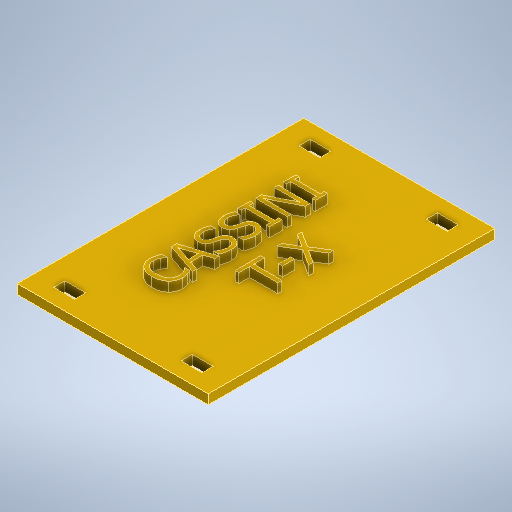
# Autodesk Inventor part: au-dessus hélice
Saved by Autodesk Inventor 2026.2 (Build 302298010, 298A)
## iProperties
Created: 2026-04-02
Part Number: au-dessus hélice
Material: Générique
Document SubType Name: Modeling
Designer: Genon
Density: 1 g/cm^3
Appearance: Or
Author: Genon
Autodesk Inventor part; units mm, degrees
ref_plane "YZ Plane" through (0, 0, 0) normal (1, 0, 0) x (0, 1, 0)
ref_plane "XZ Plane" through (0, 0, 0) normal (0, 1, 0) x (-1, 0, 0)
ref_plane "XY Plane" through (0, 0, 0) normal (0, 0, 1) x (1, 0, 0)
sketch "Esquisse1" plane through (0, 0, 0) normal (0, 1, 0) x (-1, 0, 0)
  line L0 (0, 0) -> (60, 0)
  line L1 (60, 0) -> (60, -90)
  line L2 (60, -90) -> (0, -90)
  line L3 (0, -90) -> (0, 0)
  dimension "d0" = 60
  dimension "d1" = 90
  constraints: 8 end point, 2 parallel, 1 horizontal, 1 perpendicular
  measures "d0" distance of L1.end L2.end
  measures "d1" distance of L0.end L1.end
extrude "Extrusion1" add sketch "Esquisse1" along normal blind 3
sketch "Esquisse3" plane through (0, 3, 0) normal (0, 1, 0) x (1, 0, 0)
  line L0 (-60, 0) -> (0, 0) projected
  line L1 (-30, 0) -> (-30, 90)
  line L2 (0, 90) -> (-60, 90) projected
  line L3 (-30, 45) -> (-60, 45)
  line L4 (-60, 0) -> (-60, 5)
  line L5 (-60, 90) -> (-60, 0) projected
  line L6 (-60, 5) -> (-53, 5)
  line L7 (-53, 5) -> (-47, 5)
  line L8 (-47, 5) -> (-47, 8)
  line L9 (-47, 8) -> (-53, 8)
  line L10 (-53, 8) -> (-53, 5)
  line L11 (-53, 85) -> (-47, 85)
  line L12 (-47, 85) -> (-47, 82)
  line L13 (-47, 82) -> (-53, 82)
  line L14 (-53, 82) -> (-53, 85)
  line L15 (-7, 5) -> (-13, 5)
  line L16 (-13, 5) -> (-13, 8)
  line L17 (-13, 8) -> (-7, 8)
  line L18 (-7, 8) -> (-7, 5)
  line L19 (-7, 82) -> (-7, 85)
  line L20 (-13, 82) -> (-7, 82)
  line L21 (-7, 85) -> (-13, 85)
  line L22 (-13, 85) -> (-13, 82)
  line L23 (-53, 8) -> (-53.25, 8)
  line L24 (-53.25, 8) -> (-53.25, 4.75)
  line L25 (-53.25, 4.75) -> (-53, 4.75)
  line L26 (-53, 4.75) -> (-53, 8)
  line L27 (-47, 4.75) -> (-46.75, 4.75)
  line L28 (-46.75, 4.75) -> (-46.75, 8.25)
  line L29 (-46.75, 8.25) -> (-47, 8.25)
  line L30 (-47, 8.25) -> (-47, 4.75)
  line L31 (-47, 8.25) -> (-53.25, 8.25)
  line L32 (-53.25, 8.25) -> (-53.25, 8)
  line L33 (-53.25, 8) -> (-47, 8)
  line L34 (-47, 8) -> (-47, 8.25)
  line L35 (-53, 4.75) -> (-47, 4.75)
  line L36 (-47, 4.75) -> (-47, 5)
  line L37 (-47, 5) -> (-53, 5)
  line L38 (-53, 5) -> (-53, 4.75)
  line L39 (-53.25, 82) -> (-53.25, 85.25)
  line L40 (-53.25, 85.25) -> (-53, 85.25)
  line L41 (-47, 85.25) -> (-46.75, 85.25)
  line L42 (-46.75, 85.25) -> (-46.75, 81.75)
  line L43 (-46.75, 81.75) -> (-47, 81.75)
  line L44 (-47, 81.75) -> (-53.25, 81.75)
  line L45 (-53.25, 81.75) -> (-53.25, 82)
  line L46 (-53, 85.25) -> (-47, 85.25)
  line L47 (-6.75, 8) -> (-6.75, 4.75)
  line L48 (-6.75, 4.75) -> (-7, 4.75)
  line L49 (-13, 4.75) -> (-13.25, 4.75)
  line L50 (-13.25, 4.75) -> (-13.25, 8.25)
  line L51 (-13.25, 8.25) -> (-13, 8.25)
  line L52 (-13, 8.25) -> (-6.75, 8.25)
  line L53 (-6.75, 8.25) -> (-6.75, 8)
  line L54 (-7, 4.75) -> (-13, 4.75)
  line L55 (-6.75, 82) -> (-6.75, 85.25)
  line L56 (-6.75, 81.75) -> (-6.75, 82)
  line L57 (-13, 81.75) -> (-6.75, 81.75)
  line L58 (-13.25, 81.75) -> (-13, 81.75)
  line L59 (-13.25, 85.25) -> (-13.25, 81.75)
  line L60 (-13, 85.25) -> (-13.25, 85.25)
  line L61 (-7, 85.25) -> (-13, 85.25)
  line L62 (-6.75, 85.25) -> (-7, 85.25)
  dimension "d13" = 5
  dimension "d14" = 7
  dimension "d15" = 6
  dimension "d16" = 3
  dimension "d21" = 0.25
  dimension "d22" = 3.25
  dimension "d23" = 0.25
  dimension "d24" = 3.5
  constraints: 120 end point, 39 symmetric about line, 8 parallel, 8 perpendicular, 6 point on line, 5 horizontal, 3 midpoint
  measures "d13" distance of L0.start L4.end
  measures "d14" distance of L4.end L6.end
  measures "d15" distance of L6.end L7.end
  measures "d16" distance of L7.end L8.end
  measures "d21" distance of L25.end L24.end
  measures "d22" distance of L24.end L23.end
  measures "d23" distance of L29.end L28.end
  measures "d24" distance of L28.end L27.end
extrude "Extrusion2" cut sketch "Esquisse3" against normal through all contours L24 L23 L10 L6 | L6 L26 L25 L24 | L10 L9 L8 L7 | L7 L30 L35 L26 | L32 L31 L30 L9 L23 | L8 L30 L29 L28 L27 | L11 L12 L13 L14 | L15 L16 L17 L18 | L20 L22 L21 L19 | L39 L40 L46 L41 L42 L43 L44 L45 | L47 L48 L54 L49 L50 L51 L52 L53 | L56 L57 L58 L59 L60 L61 L62 L55
sketch "Esquisse4" plane through (0, 3, 0) normal (0, 1, 0) x (1, 0, 0)
  line L0 (-45.4887, 21.9491) -> (-45.4887, 68.6531) construction
  line L1 (-45.4887, 68.6531) -> (-13.8502, 68.6531) construction
  line L2 (-13.8502, 68.6531) -> (-13.8502, 21.9491) construction
  line L3 (-13.8502, 21.9491) -> (-45.4887, 21.9491) construction
  spline S0 degree 2 poles (-32.6344, 24.588) (-32.6344, 23.6155) (-33.2908, 21.9705) (-33.9472, 21.3708) knots 0 0 0 1 2 2 2
  spline S1 degree 2 poles (-33.9472, 21.3708) (-34.5955, 20.7711) (-36.5404, 20.1147) (-37.8045, 20.1147) knots 0 0 0 1 2 2 2
  spline S2 degree 2 poles (-37.8045, 20.1147) (-39.0606, 20.1147) (-40.9245, 20.7549) (-41.6133, 21.3627) knots 0 0 0 1 2 2 2
  spline S3 degree 2 poles (-41.6133, 21.3627) (-42.2859, 21.9624) (-42.9909, 23.5993) (-42.9909, 24.6123) knots 0 0 0 1 2 2 2
  spline S4 degree 2 poles (-42.9909, 24.6123) (-42.9909, 25.1147) (-42.8451, 25.998) (-42.7316, 26.3708) knots 0 0 0 1 2 2 2
  spline S5 degree 2 poles (-42.7316, 26.3708) (-42.6263, 26.6949) (-42.3264, 27.3675) (-42.1481, 27.6998) knots 0 0 0 1 2 2 2
  line L4 (-42.1481, 27.6998) -> (-40.5436, 27.6998)
  line L5 (-40.5436, 27.6998) -> (-40.5436, 27.5945)
  spline S6 degree 2 poles (-40.5436, 27.5945) (-40.7057, 27.4162) (-41.1595, 26.8651) (-41.3783, 26.468) knots 0 0 0 1 2 2 2
  spline S7 degree 2 poles (-41.3783, 26.468) (-41.589, 26.0872) (-41.8564, 25.1876) (-41.8564, 24.6042) knots 0 0 0 1 2 2 2
  spline S8 degree 2 poles (-41.8564, 24.6042) (-41.8564, 23.964) (-41.3297, 22.8214) (-40.8272, 22.3919) knots 0 0 0 1 2 2 2
  spline S9 degree 2 poles (-40.8272, 22.3919) (-40.3167, 21.9705) (-38.7689, 21.5005) (-37.8045, 21.5005) knots 0 0 0 1 2 2 2
  spline S10 degree 2 poles (-37.8045, 21.5005) (-36.7754, 21.5005) (-35.2924, 21.9948) (-34.7819, 22.4243) knots 0 0 0 1 2 2 2
  spline S11 degree 2 poles (-34.7819, 22.4243) (-34.2875, 22.8457) (-33.7851, 23.9721) (-33.7851, 24.6042) knots 0 0 0 1 2 2 2
  spline S12 degree 2 poles (-33.7851, 24.6042) (-33.7851, 25.1795) (-34.0687, 26.1601) (-34.2794, 26.541) knots 0 0 0 1 2 2 2
  spline S13 degree 2 poles (-34.2794, 26.541) (-34.4901, 26.9056) (-34.9277, 27.4486) (-35.0817, 27.6026) knots 0 0 0 1 2 2 2
  line L6 (-35.0817, 27.6026) -> (-35.0817, 27.6998)
  line L7 (-35.0817, 27.6998) -> (-33.4934, 27.6998)
  spline S14 degree 2 poles (-33.4934, 27.6998) (-33.3394, 27.3675) (-33.0558, 26.7841) (-32.9261, 26.3708) knots 0 0 0 1 2 2 2
  spline S15 degree 2 poles (-32.9261, 26.3708) (-32.7802, 25.9332) (-32.6344, 25.1876) (-32.6344, 24.588) knots 0 0 0 1 2 2 2
  line L8 (-32.8127, 27.8619) -> (-42.8127, 31.233)
  line L9 (-42.8127, 31.233) -> (-42.8127, 32.87)
  line L10 (-42.8127, 32.87) -> (-32.8127, 36.2411)
  line L11 (-32.8127, 36.2411) -> (-32.8127, 34.8392)
  line L12 (-32.8127, 34.8392) -> (-35.6084, 33.9316)
  line L13 (-35.6084, 33.9316) -> (-35.6084, 30.1147)
  line L14 (-35.6084, 30.1147) -> (-32.8127, 29.2071)
  line L15 (-32.8127, 29.2071) -> (-32.8127, 27.8619)
  line L16 (-36.743, 33.5669) -> (-41.4512, 32.0191)
  line L17 (-41.4512, 32.0191) -> (-36.743, 30.4794)
  line L18 (-36.743, 30.4794) -> (-36.743, 33.5669)
  spline S16 degree 2 poles (-32.6344, 39.9769) (-32.6344, 38.891) (-33.0882, 37.3675) (-33.4123, 36.6949) knots 0 0 0 1 2 2 2
  line L19 (-33.4123, 36.6949) -> (-35.0817, 36.6949)
  line L20 (-35.0817, 36.6949) -> (-35.0817, 36.7922)
  spline S17 degree 2 poles (-35.0817, 36.7922) (-34.4658, 37.4486) (-33.7851, 39.1099) (-33.7851, 39.8797) knots 0 0 0 1 2 2 2
  spline S18 degree 2 poles (-33.7851, 39.8797) (-33.7851, 40.9818) (-34.7008, 42.1082) (-35.4545, 42.1082) knots 0 0 0 1 2 2 2
  spline S19 degree 2 poles (-35.4545, 42.1082) (-36.0541, 42.1082) (-36.7997, 41.5167) (-36.9861, 40.8765) knots 0 0 0 1 2 2 2
  spline S20 degree 2 poles (-36.9861, 40.8765) (-37.1157, 40.4146) (-37.294, 39.6447) (-37.4399, 39.0693) knots 0 0 0 1 2 2 2
  spline S21 degree 2 poles (-37.4399, 39.0693) (-37.5776, 38.5507) (-37.9909, 37.7322) (-38.3232, 37.4162) knots 0 0 0 1 2 2 2
  spline S22 degree 2 poles (-38.3232, 37.4162) (-38.6554, 37.1082) (-39.5468, 36.7679) (-40.1303, 36.7679) knots 0 0 0 1 2 2 2
  spline S23 degree 2 poles (-40.1303, 36.7679) (-41.3459, 36.7679) (-42.9909, 38.6641) (-42.9909, 40.1309) knots 0 0 0 1 2 2 2
  spline S24 degree 2 poles (-42.9909, 40.1309) (-42.9909, 40.9737) (-42.6587, 42.4648) (-42.3426, 43.105) knots 0 0 0 1 2 2 2
  line L21 (-42.3426, 43.105) -> (-40.7543, 43.105)
  line L22 (-40.7543, 43.105) -> (-40.7543, 43.0077)
  spline S25 degree 2 poles (-40.7543, 43.0077) (-41.1919, 42.5296) (-41.8402, 41.0385) (-41.8402, 40.2201) knots 0 0 0 1 2 2 2
  spline S26 degree 2 poles (-41.8402, 40.2201) (-41.8402, 39.2962) (-40.9731, 38.1536) (-40.2681, 38.1536) knots 0 0 0 1 2 2 2
  spline S27 degree 2 poles (-40.2681, 38.1536) (-39.636, 38.1536) (-38.8823, 38.8262) (-38.7122, 39.4583) knots 0 0 0 1 2 2 2
  spline S28 degree 2 poles (-38.7122, 39.4583) (-38.5987, 39.8797) (-38.307, 41.1034) (-38.1854, 41.5086) knots 0 0 0 1 2 2 2
  spline S29 degree 2 poles (-38.1854, 41.5086) (-37.8694, 42.5377) (-36.5971, 43.494) (-35.6652, 43.494) knots 0 0 0 1 2 2 2
  spline S30 degree 2 poles (-35.6652, 43.494) (-35.0736, 43.494) (-33.9391, 43.0158) (-33.542, 42.5863) knots 0 0 0 1 2 2 2
  spline S31 degree 2 poles (-33.542, 42.5863) (-33.1044, 42.1082) (-32.6344, 40.8927) (-32.6344, 39.9769) knots 0 0 0 1 2 2 2
  spline S32 degree 2 poles (-32.6344, 47.635) (-32.6344, 46.5491) (-33.0882, 45.0256) (-33.4123, 44.353) knots 0 0 0 1 2 2 2
  line L23 (-33.4123, 44.353) -> (-35.0817, 44.353)
  line L24 (-35.0817, 44.353) -> (-35.0817, 44.4502)
  spline S33 degree 2 poles (-35.0817, 44.4502) (-34.4658, 45.1066) (-33.7851, 46.7679) (-33.7851, 47.5377) knots 0 0 0 1 2 2 2
  spline S34 degree 2 poles (-33.7851, 47.5377) (-33.7851, 48.6398) (-34.7008, 49.7663) (-35.4545, 49.7663) knots 0 0 0 1 2 2 2
  spline S35 degree 2 poles (-35.4545, 49.7663) (-36.0541, 49.7663) (-36.7997, 49.1747) (-36.9861, 48.5345) knots 0 0 0 1 2 2 2
  spline S36 degree 2 poles (-36.9861, 48.5345) (-37.1157, 48.0726) (-37.294, 47.3027) (-37.4399, 46.7274) knots 0 0 0 1 2 2 2
  spline S37 degree 2 poles (-37.4399, 46.7274) (-37.5776, 46.2087) (-37.9909, 45.3902) (-38.3232, 45.0742) knots 0 0 0 1 2 2 2
  spline S38 degree 2 poles (-38.3232, 45.0742) (-38.6554, 44.7663) (-39.5468, 44.4259) (-40.1303, 44.4259) knots 0 0 0 1 2 2 2
  spline S39 degree 2 poles (-40.1303, 44.4259) (-41.3459, 44.4259) (-42.9909, 46.3222) (-42.9909, 47.7889) knots 0 0 0 1 2 2 2
  spline S40 degree 2 poles (-42.9909, 47.7889) (-42.9909, 48.6317) (-42.6587, 50.1228) (-42.3426, 50.763) knots 0 0 0 1 2 2 2
  line L25 (-42.3426, 50.763) -> (-40.7543, 50.763)
  line L26 (-40.7543, 50.763) -> (-40.7543, 50.6658)
  spline S41 degree 2 poles (-40.7543, 50.6658) (-41.1919, 50.1876) (-41.8402, 48.6966) (-41.8402, 47.8781) knots 0 0 0 1 2 2 2
  spline S42 degree 2 poles (-41.8402, 47.8781) (-41.8402, 46.9543) (-40.9731, 45.8116) (-40.2681, 45.8116) knots 0 0 0 1 2 2 2
  spline S43 degree 2 poles (-40.2681, 45.8116) (-39.636, 45.8116) (-38.8823, 46.4842) (-38.7122, 47.1163) knots 0 0 0 1 2 2 2
  spline S44 degree 2 poles (-38.7122, 47.1163) (-38.5987, 47.5377) (-38.307, 48.7614) (-38.1854, 49.1666) knots 0 0 0 1 2 2 2
  spline S45 degree 2 poles (-38.1854, 49.1666) (-37.8694, 50.1958) (-36.5971, 51.152) (-35.6652, 51.152) knots 0 0 0 1 2 2 2
  spline S46 degree 2 poles (-35.6652, 51.152) (-35.0736, 51.152) (-33.9391, 50.6739) (-33.542, 50.2444) knots 0 0 0 1 2 2 2
  spline S47 degree 2 poles (-33.542, 50.2444) (-33.1044, 49.7663) (-32.6344, 48.5507) (-32.6344, 47.635) knots 0 0 0 1 2 2 2
  line L27 (-32.8127, 55.9899) -> (-32.8127, 52.1163)
  line L28 (-32.8127, 52.1163) -> (-33.8337, 52.1163)
  line L29 (-33.8337, 52.1163) -> (-33.8337, 53.3886)
  line L30 (-33.8337, 53.3886) -> (-41.7916, 53.3886)
  line L31 (-41.7916, 53.3886) -> (-41.7916, 52.1163)
  line L32 (-41.7916, 52.1163) -> (-42.8127, 52.1163)
  line L33 (-42.8127, 52.1163) -> (-42.8127, 55.9899)
  line L34 (-42.8127, 55.9899) -> (-41.7916, 55.9899)
  line L35 (-41.7916, 55.9899) -> (-41.7916, 54.7176)
  line L36 (-41.7916, 54.7176) -> (-33.8337, 54.7176)
  line L37 (-33.8337, 54.7176) -> (-33.8337, 55.9899)
  line L38 (-33.8337, 55.9899) -> (-32.8127, 55.9899)
  line L39 (-32.8127, 64.7906) -> (-32.8127, 63.2995)
  line L40 (-32.8127, 63.2995) -> (-41.435, 58.8748)
  line L41 (-41.435, 58.8748) -> (-32.8127, 58.8748)
  line L42 (-32.8127, 58.8748) -> (-32.8127, 57.635)
  line L43 (-32.8127, 57.635) -> (-42.8127, 57.635)
  line L44 (-42.8127, 57.635) -> (-42.8127, 59.5231)
  line L45 (-42.8127, 59.5231) -> (-34.8953, 63.5507)
  line L46 (-34.8953, 63.5507) -> (-42.8127, 63.5507)
  line L47 (-42.8127, 63.5507) -> (-42.8127, 64.7906)
  line L48 (-42.8127, 64.7906) -> (-32.8127, 64.7906)
  line L49 (-32.8127, 70.3011) -> (-32.8127, 66.4275)
  line L50 (-32.8127, 66.4275) -> (-33.8337, 66.4275)
  line L51 (-33.8337, 66.4275) -> (-33.8337, 67.6998)
  line L52 (-33.8337, 67.6998) -> (-41.7916, 67.6998)
  line L53 (-41.7916, 67.6998) -> (-41.7916, 66.4275)
  line L54 (-41.7916, 66.4275) -> (-42.8127, 66.4275)
  line L55 (-42.8127, 66.4275) -> (-42.8127, 70.3011)
  line L56 (-42.8127, 70.3011) -> (-41.7916, 70.3011)
  line L57 (-41.7916, 70.3011) -> (-41.7916, 69.0288)
  line L58 (-41.7916, 69.0288) -> (-33.8337, 69.0288)
  line L59 (-33.8337, 69.0288) -> (-33.8337, 70.3011)
  line L60 (-33.8337, 70.3011) -> (-32.8127, 70.3011)
  line L61 (-16.3479, 38.1455) -> (-25.1648, 38.1455)
  line L62 (-25.1648, 38.1455) -> (-25.1648, 34.7906)
  line L63 (-25.1648, 34.7906) -> (-26.3479, 34.7906)
  line L64 (-26.3479, 34.7906) -> (-26.3479, 42.8295)
  line L65 (-26.3479, 42.8295) -> (-25.1648, 42.8295)
  line L66 (-25.1648, 42.8295) -> (-25.1648, 39.4745)
  line L67 (-25.1648, 39.4745) -> (-16.3479, 39.4745)
  line L68 (-16.3479, 39.4745) -> (-16.3479, 38.1455)
  line L69 (-20.1161, 47.2217) -> (-20.1161, 43.4372)
  line L70 (-20.1161, 43.4372) -> (-21.3317, 43.4372)
  line L71 (-21.3317, 43.4372) -> (-21.3317, 47.2217)
  line L72 (-21.3317, 47.2217) -> (-20.1161, 47.2217)
  line L73 (-16.3479, 55.7468) -> (-16.3479, 54.2233)
  line L74 (-16.3479, 54.2233) -> (-20.3349, 51.7922)
  line L75 (-20.3349, 51.7922) -> (-16.3479, 49.3124)
  line L76 (-16.3479, 49.3124) -> (-16.3479, 47.8781)
  line L77 (-16.3479, 47.8781) -> (-21.356, 51.0628)
  line L78 (-21.356, 51.0628) -> (-26.3479, 47.9753)
  line L79 (-26.3479, 47.9753) -> (-26.3479, 49.4988)
  line L80 (-26.3479, 49.4988) -> (-22.4338, 51.8813)
  line L81 (-22.4338, 51.8813) -> (-26.3479, 54.3124)
  line L82 (-26.3479, 54.3124) -> (-26.3479, 55.7468)
  line L83 (-26.3479, 55.7468) -> (-21.4208, 52.6188)
  line L84 (-21.4208, 52.6188) -> (-16.3479, 55.7468)
  point P0 (0, 0)
  constraints: 2 other
extrude "Extrusion3" add sketch "Esquisse4" along normal blind 3
